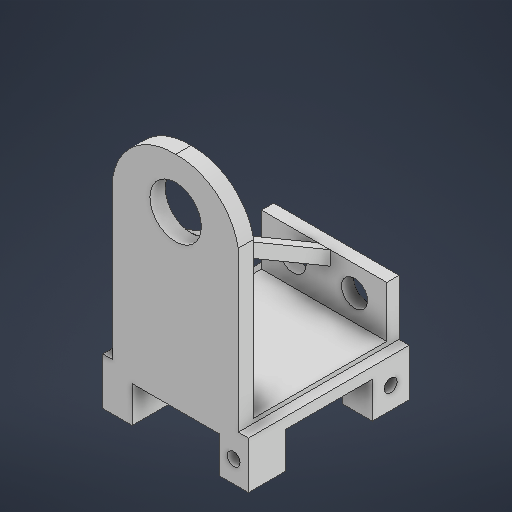
# Autodesk Inventor part: Transmitter + Reciever
Saved by Autodesk Inventor 2027 (Build 310192060, 192F)
## iProperties
Created: 2026-05-19
Part Number: Transmitter + Reciever
Material: Generic
Document SubType Name: Modeling
Designer: blaze
Density: 1 g/cm^3
Appearance: Default
Author: blaze
Autodesk Inventor part; units mm, degrees
ref_plane "YZ Plane" through (0, 0, 0) normal (1, 0, 0) x (0, 1, 0)
ref_plane "XZ Plane" through (0, 0, 0) normal (0, 1, 0) x (-1, 0, 0)
sketch "Sketch1" plane through (0, 0, 0) normal (0, 0, 1) x (1, 0, 0)
  line L0 (0, 0) -> (38.989, 0)
  line L1 (0, 8.1026) -> (0, 61.0616)
  line L2 (38.989, 8.1026) -> (38.989, 61.0616)
  arc A0 (19.4945, 76.6064) -> (0, 61.0616) centre (18.7276, 57.5718) ccw
  arc A1 (38.989, 61.0616) -> (19.4945, 76.6064) centre (20.2614, 57.5718) ccw
  line L3 (0, 8.1026) -> (38.989, 8.1026)
  line L4 (0, 61.0616) -> (38.989, 61.0616)
  dimension "d3" = 19.05
  dimension "d4" = 19.05
  constraints: 10 end point, 4 point on circle, 2 centre point, 2 horizontal, 2 vertical, 1 perpendicular
  measures "d3" radius of A0
  measures "d4" radius of A1
extrude "Extrusion1" add sketch "Sketch1" against normal blind 4.8006
sketch "Sketch2" plane through (0, 0, 0) normal (0, 0, 1) x (1, 0, 0)
  line L0 (38.989, 8.1026) -> (0, 8.1026) projected
  line L1 (38.989, 61.0616) -> (38.989, 8.1026) projected
  line L2 (5.9944, 8.1026) -> (32.9946, 8.1026)
  line L3 (38.989, 11.5157) -> (38.989, 12.8778)
  line L4 (38.989, 12.8778) -> (0, 12.8778)
  line L5 (0, 12.8778) -> (0, 11.5157)
  line L6 (5.9944, 8.1026) -> (5.9944, 0)
  line L7 (5.9944, 0) -> (0, 0)
  line L8 (32.9946, 8.1026) -> (32.9946, 0)
  line L9 (32.9946, 0) -> (38.989, 0)
  line L10 (38.989, 0) -> (42.164, 0)
  line L11 (42.164, 0) -> (42.164, 11.5157)
  line L12 (42.164, 11.5157) -> (38.989, 11.5157)
  line L13 (38.989, 12.8778) -> (38.989, 11.5157)
  line L14 (0, 0) -> (-3.175, 0)
  line L15 (-3.175, 0) -> (-3.175, 11.5157)
  line L16 (-3.175, 11.5157) -> (0, 11.5157)
  constraints: 30 end point, 4 perpendicular, 4 point on line, 3 parallel, 2 horizontal
extrude "Extrusion2" add sketch "Sketch2" against normal blind 50.0126 contours L0 L6 L7 L14 L15 L16 L5 L4 L1
sketch "Sketch3" plane through (0, 0, -50.0126) normal (0, 0, -1) x (-1, 0, 0)
  line L0 (-38.989, 12.8778) -> (0, 12.8778) projected
  line L1 (-4.4958, 12.8778) -> (-34.4932, 12.8778)
  line L2 (-34.4932, 28.7528) -> (-4.4958, 28.7528)
  line L3 (-38.989, 8.1026) -> (-38.989, 61.0616) projected
  circle A0 centre (-28.9433, 20.8153) radius 4.0513
  circle A1 centre (-9.8425, 20.8153) radius 4.0513
  line L4 (-34.4932, 12.8778) -> (-38.989, 12.8778)
  line L5 (-38.989, 12.8778) -> (-38.989, 28.7528)
  line L6 (-38.989, 28.7528) -> (-34.4932, 28.7528)
  line L7 (-4.4958, 28.7528) -> (0, 28.7528)
  line L8 (0, 12.8778) -> (0, 61.0616) projected
  line L9 (0, 28.7528) -> (0, 12.8778)
  line L10 (0, 12.8778) -> (-4.4958, 12.8778)
  point P0 (0, 0)
  point P1 (-38.989, 0)
  dimension "d17" = 8.1026
  dimension "d19" = 8.1026
  constraints: 16 end point, 3 point on line, 2 centre point, 2 collinear, 2 horizontal, 2 perpendicular, 1 parallel
  measures "d17" diameter of A0
  measures "d19" diameter of A1
extrude "Extrusion3" add sketch "Sketch3" against normal blind 3.81
ref_plane "Work Plane1" through (19.4945, 61.0616, 0) normal (1, 0, 0) x (0, 0, -1)
sketch "Sketch6" plane through (0, 0, 0) normal (0, 0, 1) x (1, 0, 0)
  line L0 (0, 61.0616) -> (0, 0) projected
  arc A0 (38.989, 61.0616) -> (19.4945, 76.6064) centre (20.2614, 57.5718) ccw projected
  circle A1 centre (19.4945, 61.0616) radius 8
  dimension "d22" = 16
  constraints: 1 centre point
  measures "d22" diameter of A1
extrude "Extrusion4" cut sketch "Sketch6" against normal blind 5.3975
sketch "Sketch7" plane through (19.4945, 61.0616, 0) normal (1, 0, 0) x (0, 0, -1)
  line L0 (0, -8) -> (4.8006, -8) projected
  line L1 (4.8006, -8) -> (46.2026, -32.3088)
  line L2 (46.2026, -32.3088) -> (46.2026, -48.1838)
  line L3 (4.8006, 0) -> (4.8006, -48.1838) projected
  line L4 (46.2026, -44.2976) -> (46.2026, -36.195) projected
  line L5 (46.2026, -36.727) -> (4.8006, -12.4182)
  point P0 (0, -61.0616)
  constraints: 6 end point, 3 point on line, 1 vertical
extrude "Extrusion5" add sketch "Sketch7" along normal mid plane 3.81
sketch "Sketch11" plane through (38.989, 61.0616, 0) normal (1, 0, 0) x (0, 0, -1)
  line L0 (0, -61.0616) -> (50.0126, -61.0616) projected
  line L1 (50.0126, -48.1838) -> (50.0126, -61.0616) projected
  circle A0 centre (25.0063, -57.2836) radius 2
  dimension "d54" = 4
  constraints: 1 centre point
  measures "d54" diameter of A0
extrude "Extrusion8" cut sketch "Sketch11" against normal blind 7.9375
extrude "Extrusion9" add sketch "Sketch2" against normal up to surface (50.0126 mm away) contours L1 L12 L11 L10 L9 L8 L0
sketch "Sketch12" plane through (42.164, 0, 0) normal (1, 0, 0) x (0, 0, -1)
  line L0 (0, 0) -> (50.0126, 0) projected
  line L1 (25.0063, 8.1026) -> (11.5062, 8.1026)
  line L2 (11.5062, 8.1026) -> (11.5062, 0)
  line L3 (25.0063, 8.1026) -> (38.5064, 8.1026)
  line L4 (0, 8.1026) -> (50.0126, 8.1026) projected
  line L5 (38.5064, 8.1026) -> (38.5064, 0)
  line L6 (11.5062, 0) -> (38.5064, 0)
  dimension "d63" = 13.5001
  dimension "d64" = 13.5001
  constraints: 10 end point, 3 point on line, 2 perpendicular, 1 collinear
  measures "d63" distance of L1.start L1.end
  measures "d64" distance of L1.start L3.end
extrude "Extrusion10" cut sketch "Sketch12" against normal up to surface (45.339 mm away)
sketch "Sketch13" plane through (0, 0, 0) normal (0, 0, 1) x (1, 0, 0)
  circle A0 centre (37.5793, 3.6) radius 2
  line L0 (32.9946, 0) -> (42.164, 0) projected
  line L1 (37.5793, 0) -> (37.5793, 1.6)
  line L2 (37.5793, 0) -> (39.1793, 0) construction
  point P0 (0, 0)
  dimension "d67" = 4
  dimension "d68" = 1.6
  dimension "d69" = 90
  constraints: 4 end point, 1 centre point, 1 horizontal, 1 midpoint, 1 perpendicular, 1 vertical
  measures "d67" diameter of A0
  measures "d68" distance of L1.start L1.end
  measures "d69" angle of L2 L1
extrude "Extrusion11" cut sketch "Sketch13" against normal up to surface (11.5062 mm away)
sketch "Sketch14" plane through (42.164, 0, 0) normal (1, 0, 0) x (0, 0, -1)
  circle A0 centre (44.2595, 3.6) radius 2
  point P0 (0, 0)
  point P1 (38.5064, 0)
  point P2 (50.0126, 0)
  dimension "d73" = 4
  constraints: 1 centre point
  measures "d73" diameter of A0
extrude "Extrusion12" cut sketch "Sketch14" against normal up to surface (45.339 mm away)
sketch "Sketch15" plane through (0, 0, 0) normal (0, 0, 1) x (1, 0, 0)
  line L0 (-3.175, 0) -> (5.9944, 0) projected
  line L1 (-3.175, 0) -> (5.9944, 0)
  line L2 (5.9944, 0) -> (5.9944, -3.175)
  line L3 (5.9944, -3.175) -> (-3.175, -3.175)
  line L4 (-3.175, -3.175) -> (-3.175, 0)
  line L5 (32.9946, 0) -> (42.164, 0) projected
  line L6 (32.9946, 0) -> (42.164, 0)
  line L7 (42.164, 0) -> (42.164, -3.175)
  line L8 (42.164, -3.175) -> (32.9946, -3.175)
  line L9 (32.9946, -3.175) -> (32.9946, 0)
  point P0 (0, 0)
  dimension "d76" = 3.175
  dimension "d77" = 3.175
  constraints: 16 end point, 4 parallel, 2 horizontal, 2 perpendicular
  measures "d76" distance of L1.end L2.end
  measures "d77" distance of L6.end L7.end
extrude "Extrusion13" add sketch "Sketch15" against normal up to surface (50.0126 mm away)
sketch "Sketch16" plane through (-3.175, 11.5157, -50.0126) normal (-1, 0, 0) x (0, 0, 1)
  line L0 (38.5064, -11.5157) -> (11.5062, -11.5157) projected
  line L1 (38.5064, -11.5157) -> (38.5064, -14.6907)
  line L2 (50.0126, -14.6907) -> (0, -14.6907) projected
  line L3 (11.5062, -11.5157) -> (38.5064, -11.5157)
  line L4 (38.5064, -11.5157) -> (38.5064, -14.6907)
  line L5 (38.5064, -14.6907) -> (11.5062, -14.6907)
  line L6 (11.5062, -14.6907) -> (11.5062, -11.5157)
  point P0 (50.0126, -11.5157)
  constraints: 10 end point, 2 parallel, 1 horizontal, 1 perpendicular, 1 point on line, 1 vertical
extrude "Extrusion14" cut sketch "Sketch16" against normal up to surface (45.339 mm away)
body "Solid1"
